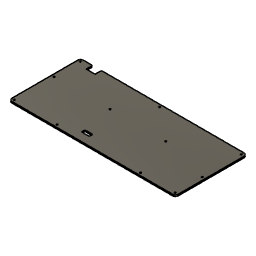
rowlow52he-bottomalumi v1 (Autodesk Fusion 360 design; units mm, degrees)
Autodesk Fusion 360 part; units mm, degrees
sketch "スケッチ1" plane through (0, 0, 0) normal (0, 0, 1) x (1, 0, 0)
  spline S0 degree 3 poles (61.2138, -44.8309) (61.2138, -44.2739) (60.7548, -43.8149) (60.1978, -43.8149) knots 0 0 0 0 1 1 1 1
  line L0 (147.3196, -135.6356) -> (137.7946, -135.6356)
  spline S1 degree 3 poles (137.0326, -134.8736) (137.0326, -135.2916) (137.3766, -135.6356) (137.7946, -135.6356) knots 0 0 0 0 1 1 1 1
  line L1 (47.8149, -147.9546) -> (282.0642, -147.9546)
  line L2 (61.2138, -52.9589) -> (74.1678, -52.9589)
  spline S2 degree 3 poles (75.4378, -43.8149) (74.7408, -43.8149) (74.1678, -44.3879) (74.1678, -45.0849) knots 0 0 0 0 1 1 1 1
  spline S3 degree 3 poles (148.2086, -131.4446) (148.2086, -131.0266) (147.8646, -130.6826) (147.4466, -130.6826) knots 0 0 0 0 1 1 1 1
  spline S4 degree 3 poles (47.8149, -43.8149) (45.6209, -43.8149) (43.8149, -45.6209) (43.8149, -47.8149) knots 0 0 0 0 1 1 1 1
  spline S5 degree 3 poles (137.5406, -130.6826) (137.2616, -130.6826) (137.0326, -130.9116) (137.0326, -131.1906) knots 0 0 0 0 1 1 1 1
  line L3 (148.2086, -131.4446) -> (148.2086, -134.7466)
  spline S6 degree 3 poles (286.0642, -47.8149) (286.0642, -45.6209) (284.2582, -43.8149) (282.0642, -43.8149) knots 0 0 0 0 1 1 1 1
  line L4 (74.1678, -52.9589) -> (74.1678, -45.0849)
  line L5 (43.8149, -143.9546) -> (43.8149, -47.8149)
  spline S7 degree 3 poles (147.3196, -135.6356) (147.8076, -135.6356) (148.2086, -135.2346) (148.2086, -134.7466) knots 0 0 0 0 1 1 1 1
  spline S8 degree 3 poles (43.8149, -143.9546) (43.8149, -146.1486) (45.6209, -147.9546) (47.8149, -147.9546) knots 0 0 0 0 1 1 1 1
  line L6 (61.2138, -44.8309) -> (61.2138, -52.9589)
  line L7 (137.5406, -130.6826) -> (147.4466, -130.6826)
  line L8 (286.0642, -143.9546) -> (286.0642, -47.8149)
  line L9 (47.8149, -43.8149) -> (60.1978, -43.8149)
  spline S9 degree 3 poles (282.0642, -147.9546) (284.2582, -147.9546) (286.0642, -146.1486) (286.0642, -143.9546) knots 0 0 0 0 1 1 1 1
  line L10 (137.0326, -134.8736) -> (137.0326, -131.1906)
  line L11 (282.0642, -43.8149) -> (75.4378, -43.8149)
  circle A0 centre (47.4979, -47.6249) radius 1.15
  circle A1 centre (231.3934, -144.1446) radius 1.15
  circle A2 centre (281.8122, -47.6249) radius 1.15
  circle A3 centre (109.9817, -144.1446) radius 1.15
  circle A4 centre (47.4979, -86.2328) radius 1.15
  circle A5 centre (129.2856, -86.2328) radius 1.15
  circle A6 centre (210.1844, -86.2328) radius 1.15
  circle A7 centre (47.4979, -144.1446) radius 1.15
  circle A8 centre (281.8122, -104.5207) radius 1.15
  circle A9 centre (281.8122, -144.1446) radius 1.15
  circle A10 centre (162.4326, -47.6249) radius 1.15
  point P0 (48.6479, -47.6249)
  point P1 (232.5434, -144.1446)
  point P2 (282.9622, -47.6249)
  point P3 (111.1317, -144.1446)
  point P4 (48.6479, -86.2328)
  point P5 (130.4356, -86.2328)
  point P6 (211.3344, -86.2328)
  point P7 (48.6479, -144.1446)
  point P8 (282.9622, -104.5207)
  point P9 (282.9622, -144.1446)
  point P10 (163.5826, -47.6249)
extrude "押し出し1" add sketch "スケッチ1" along normal blind 2
